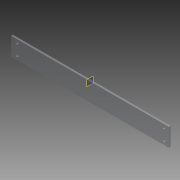
# Autodesk Inventor part: GE-13041
Saved by Autodesk Inventor 2013 (Build 170138000, 138)
## iProperties
Created: 2013-01-06
Part Number: GE-13041
Material: Polycarbonate, Clear
Document SubType Name: Modeling
Designer: Phillip
Density: 1 g/cm^3
Author: Phillip
Autodesk Inventor part; units mm, degrees
ref_plane "YZ Plane" through (0, 0, 0) normal (1, 0, 0) x (0, 1, 0)
ref_plane "XZ Plane" through (0, 0, 0) normal (0, 1, 0) x (-1, 0, 0)
ref_plane "XY Plane" through (0, 0, 0) normal (0, 0, 1) x (1, 0, 0)
sketch "Sketch1" plane through (0, 0, 0) normal (0, 0, 1) x (1, 0, 0)
  line L0 (-276.225, -31.75) -> (276.225, -31.75)
  line L1 (276.225, -31.75) -> (276.225, 31.75)
  line L2 (276.225, 31.75) -> (-276.225, 31.75)
  line L3 (-276.225, 31.75) -> (-276.225, -31.75)
  line L4 (-276.225, -31.75) -> (276.225, 31.75) construction
  line L5 (276.225, -31.75) -> (-276.225, 31.75) construction
  point P0 (0, 0)
  dimension "d0" = 552.45
  dimension "d1" = 63.5
  constraints: 12 end point, 2 midpoint, 2 parallel, 1 horizontal, 1 perpendicular
  measures "d0" distance of L2.end L1.end
  measures "d1" distance of L1.end L0.end
extrude "Extrusion1" add sketch "Sketch1" against normal blind 6.35
sketch "Sketch2" plane through (0, 0, 0) normal (0, 0, 1) x (1, 0, 0)
  line L0 (276.225, 31.75) -> (-276.225, 31.75) projected
  line L1 (-276.225, 31.75) -> (-276.225, -31.75) projected
  point P0 (0, 0)
  point P1 (-257.175, 19.05)
  point P2 (-257.175, -19.05)
  point P3 (257.175, 19.05)
  point P4 (257.175, -19.05)
  dimension "d4" = 19.05
  dimension "d5" = 12.7
  dimension "d6" = 50.8
  dimension "d8" = 533.4
  constraints: 2 horizontal alignment, 2 vertical alignment
  measures "d4" distance from line of point (-257.175, 19.05) L1
  measures "d5" distance from line of point (-257.175, 19.05) L0
  measures "d6" distance from line of point (-257.175, -19.05) L0
  measures "d8" distance from line of point (257.175, 19.05) L1
hole "Hole1" at (-257.175, 19.05, 0) at (-257.175, -19.05, 0) at (257.175, 19.05, 0) at (257.175, -19.05, 0) direction (0, 0, -1) diameter 7.874 end through all
ref_plane "Work Plane1" through (0, 31.75, 0) normal (-1, 0, 0) x (0, -1, 0)
body "Solid1"
